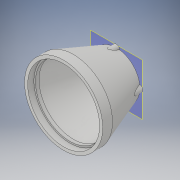
# Autodesk Inventor part: endkappen
Saved by Autodesk Inventor 2017 (Build 210142000, 142)
## iProperties
Part Number: endkappen
Material: Generisch
Document SubType Name: Modeling
Designer: Fabio
Density: 1 g/cm^3
Appearance: Vorgabe
Author: Fabio
Autodesk Inventor part; units mm, degrees
ref_plane "YZ Plane" through (0, 0, 0) normal (1, 0, 0) x (0, 1, 0)
ref_plane "XZ Plane" through (0, 0, 0) normal (0, 1, 0) x (-1, 0, 0)
ref_plane "XY Plane" through (0, 0, 0) normal (0, 0, 1) x (1, 0, 0)
sketch "Skizze2" plane through (0, 0, 0) normal (1, 0, 0) x (0, 1, 0)
  line L0 (6.2626, 25) -> (33.7374, 15)
  line L1 (33.7374, 15) -> (33.7374, 12)
  line L2 (33.7374, 12) -> (6.2626, 22)
  line L3 (0, 0) -> (48.6481, 0)
  line L4 (6.2626, 25) -> (0, 25)
  line L5 (6.2626, 22) -> (4, 22)
  line L6 (4, 22) -> (4, 23)
  line L7 (4, 23) -> (0, 23)
  line L8 (0, 0) -> (0, 23) construction
  line L9 (0, 23) -> (0, 25)
  dimension "d20" = 30
  dimension "d21" = 24
  dimension "d22" = 20
  dimension "d55" = 4
  dimension "d56" = 2
  dimension "d57" = 50
  dimension "d58" = 2.2626
  dimension "d59" = 1
  dimension "d60" = 6.2626
  constraints: 20 end point, 3 horizontal, 2 perpendicular, 1 collinear, 1 parallel, 1 vertical
  measures "d20" diameter of L0.end L3
  measures "d21" diameter of L1.end L3
  measures "d22" angle of L3 L2
  measures "d55" distance of L6.end L7.end
  measures "d56" distance of L7.end L4.end
  measures "d57" diameter of L4 L3
  measures "d58" distance of L2.end L5.end
  measures "d59" distance of L5.end L6.end
  measures "d60" distance of L0.start L4.end
revolve "Umdrehung1" add sketch "Skizze2" angle 360 about axis through (0, 0, 0) along (0, 1, 0)
ref_plane "Arbeitsebene1" through (0, 33.7374, 0) normal (0, 1, 0) x (1, 0, 0)
sketch "Skizze3" plane through (0, 33.7374, 0) normal (0, 1, 0) x (1, 0, 0)
  circle A0 centre (0, 0) radius 15 construction
  circle A1 centre (0, 0) radius 12 construction
  line L0 (0, 0) -> (0, -15) construction
  circle A2 centre (0, -15) radius 2
  circle A3 centre (15, 0) radius 2
  circle A4 centre (0, 15) radius 2
  circle A5 centre (-15, 0) radius 2
  dimension "d32" = 4
  dimension "d35" = 360
  constraints: 4 centre point, 2 end point, 1 coincident, 1 vertical, 1 vertical alignment, 10 other
  measures "d32" diameter of A2
extrude "Extrusion3" add sketch "Skizze3" against normal blind 6 separate body
combine bodies "Kombinieren1" operation type add bodies to combine 2 1
delete faces "Fläche löschen3" heal yes whole lump no faces at (-13, 28.8216, 0) (-13.7858, 27.7374, -0.0804)
delete faces "Fläche löschen4" heal yes whole lump no faces at (0, 28.8216, 13) (13, 28.8213, 0.0105) (0.0104, 28.8213, -13) (13.7858, 27.7374, -0.0804) (-0.0804, 27.7374, -13.7858) (0.2778, 27.7374, 13.79)
sketch "Skizze4" plane through (0, 33.7374, 0) normal (0, 1, 0) x (1, 0, 0)
  arc A0 (-14.8667, 1.9956) -> (-14.8667, -1.9956) centre (-15, 0) ccw projected
  arc A1 (1.9956, 14.8667) -> (-1.9956, 14.8667) centre (0, 15) ccw projected
  arc A2 (14.8667, -1.9956) -> (14.8667, 1.9956) centre (15, 0) ccw projected
  arc A3 (-1.9956, -14.8667) -> (1.9956, -14.8667) centre (0, -15) ccw projected
  point P0 (0, 0)
  constraints: 4 coincident
hole "Bohrung1" at (-15, 33.7374, 0) at (0, 33.7374, -15) at (15, 33.7374, 0) at (0, 33.7374, 15) direction (0, -1, 0) diameter 2 end through all bodies 2
